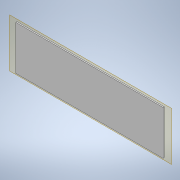
# Autodesk Inventor part: ferrite_layer_dex_laser_cut
Saved by Autodesk Inventor 2020 (Build 240168000, 168)
## iProperties
Created: 2021-01-27
Part Number: ferrite_layer_dex_laser_cut
Material: Generic
Document SubType Name: Modeling
Designer: pduy110
Density: 1 g/cm^3
Appearance: Default
Author: pduy110
Autodesk Inventor part; units mm, degrees
ref_plane "YZ Plane" through (0, 0, 0) normal (1, 0, 0) x (0, 1, 0)
ref_plane "XZ Plane" through (0, 0, 0) normal (0, 1, 0) x (-1, 0, 0)
sketch "ferrite_layer_outline_sketch" plane through (0, 0, 0) normal (0, 0, 1) x (1, 0, 0)
  line L0 (0, 150) -> (1000, 150)
  line L1 (1000, 150) -> (1000, -150)
  line L2 (1000, -150) -> (0, -150)
  line L3 (0, -150) -> (0, 150)
  line L4 (-200, 0) -> (1200, 0) projected
  line L5 (500, 150) -> (500, -150) construction
  line L6 (500, 366.8869) -> (500, -324.3455) construction
  line L7 (20, 109) -> (35, 109)
  line L8 (35, 109) -> (35, -109)
  line L9 (35, -109) -> (20, -109)
  line L10 (20, -109) -> (20, 109)
  line L11 (177.5, -109) -> (177.5, 109)
  line L12 (177.5, 109) -> (192.5, 109)
  line L13 (192.5, 109) -> (192.5, -109)
  line L14 (192.5, -109) -> (177.5, -109)
  line L15 (335, -109) -> (335, 109)
  line L16 (335, 109) -> (350, 109)
  line L17 (350, 109) -> (350, -109)
  line L18 (350, -109) -> (335, -109)
  line L19 (492.5, -109) -> (492.5, 109)
  line L20 (492.5, 109) -> (507.5, 109)
  line L21 (507.5, 109) -> (507.5, -109)
  line L22 (507.5, -109) -> (492.5, -109)
  line L23 (650, -109) -> (650, 109)
  line L24 (650, 109) -> (665, 109)
  line L25 (665, 109) -> (665, -109)
  line L26 (665, -109) -> (650, -109)
  line L27 (807.5, -109) -> (807.5, 109)
  line L28 (807.5, 109) -> (822.5, 109)
  line L29 (822.5, 109) -> (822.5, -109)
  line L30 (822.5, -109) -> (807.5, -109)
  line L31 (965, -109) -> (965, 109)
  line L32 (965, 109) -> (980, 109)
  line L33 (980, 109) -> (980, -109)
  line L34 (980, -109) -> (965, -109)
  line L35 (155, 109) -> (170, 109)
  line L36 (155, -109) -> (155, 109)
  line L37 (170, 109) -> (170, -109)
  line L38 (170, -109) -> (155, -109)
  line L39 (290, 109) -> (305, 109)
  line L40 (290, -109) -> (290, 109)
  line L41 (305, 109) -> (305, -109)
  line L42 (305, -109) -> (290, -109)
  line L43 (425, 109) -> (440, 109)
  line L44 (425, -109) -> (425, 109)
  line L45 (440, 109) -> (440, -109)
  line L46 (440, -109) -> (425, -109)
  line L47 (560, 109) -> (575, 109)
  line L48 (560, -109) -> (560, 109)
  line L49 (575, 109) -> (575, -109)
  line L50 (575, -109) -> (560, -109)
  line L51 (695, 109) -> (710, 109)
  line L52 (695, -109) -> (695, 109)
  line L53 (710, 109) -> (710, -109)
  line L54 (710, -109) -> (695, -109)
  line L55 (830, 109) -> (845, 109)
  line L56 (830, -109) -> (830, 109)
  line L57 (845, 109) -> (845, -109)
  line L58 (845, -109) -> (830, -109)
  line L59 (965, 109) -> (980, 109)
  line L60 (965, -109) -> (965, 109)
  line L61 (980, 109) -> (980, -109)
  line L62 (980, -109) -> (965, -109)
  line L63 (125, -109) -> (125, 109)
  line L64 (125, 109) -> (140, 109)
  line L65 (140, 109) -> (140, -109)
  line L66 (230, -109) -> (230, 109)
  line L67 (230, 109) -> (245, 109)
  line L68 (245, 109) -> (245, -109)
  line L69 (335, -109) -> (335, 109)
  line L70 (335, 109) -> (350, 109)
  line L71 (350, 109) -> (350, -109)
  line L72 (440, -109) -> (440, 109)
  line L73 (440, 109) -> (455, 109)
  line L74 (455, 109) -> (455, -109)
  line L75 (545, -109) -> (545, 109)
  line L76 (545, 109) -> (560, 109)
  line L77 (560, 109) -> (560, -109)
  line L78 (650, -109) -> (650, 109)
  line L79 (650, 109) -> (665, 109)
  line L80 (665, 109) -> (665, -109)
  line L81 (755, -109) -> (755, 109)
  line L82 (755, 109) -> (770, 109)
  line L83 (770, 109) -> (770, -109)
  line L84 (860, -109) -> (860, 109)
  line L85 (860, 109) -> (875, 109)
  line L86 (875, 109) -> (875, -109)
  line L87 (965, -109) -> (965, 109)
  line L88 (965, 109) -> (980, 109)
  line L89 (980, 109) -> (980, -109)
  line L90 (114.5, -109) -> (114.5, 109)
  line L91 (114.5, 109) -> (129.5, 109)
  line L92 (129.5, 109) -> (129.5, -109)
  line L93 (129.5, -109) -> (114.5, -109)
  line L94 (209, -109) -> (209, 109)
  line L95 (209, 109) -> (224, 109)
  line L96 (224, 109) -> (224, -109)
  line L97 (224, -109) -> (209, -109)
  line L98 (303.5, -109) -> (303.5, 109)
  line L99 (303.5, 109) -> (318.5, 109)
  line L100 (318.5, 109) -> (318.5, -109)
  line L101 (318.5, -109) -> (303.5, -109)
  line L102 (398, -109) -> (398, 109)
  line L103 (398, 109) -> (413, 109)
  line L104 (413, 109) -> (413, -109)
  line L105 (413, -109) -> (398, -109)
  line L106 (492.5, -109) -> (492.5, 109)
  line L107 (492.5, 109) -> (507.5, 109)
  line L108 (507.5, 109) -> (507.5, -109)
  line L109 (507.5, -109) -> (492.5, -109)
  line L110 (587, -109) -> (587, 109)
  line L111 (587, 109) -> (602, 109)
  line L112 (602, 109) -> (602, -109)
  line L113 (602, -109) -> (587, -109)
  line L114 (681.5, -109) -> (681.5, 109)
  line L115 (681.5, 109) -> (696.5, 109)
  line L116 (696.5, 109) -> (696.5, -109)
  line L117 (696.5, -109) -> (681.5, -109)
  line L118 (776, -109) -> (776, 109)
  line L119 (776, 109) -> (791, 109)
  line L120 (791, 109) -> (791, -109)
  line L121 (791, -109) -> (776, -109)
  line L122 (870.5, -109) -> (870.5, 109)
  line L123 (870.5, 109) -> (885.5, 109)
  line L124 (885.5, 109) -> (885.5, -109)
  line L125 (885.5, -109) -> (870.5, -109)
  line L126 (965, -109) -> (965, 109)
  line L127 (965, 109) -> (980, 109)
  line L128 (980, 109) -> (980, -109)
  line L129 (980, -109) -> (965, -109)
  point P0 (0, 0)
  point P1 (0, 0)
  point P2 (0, 0)
  point P3 (0, 0)
  point P4 (20, 0)
  point P5 (177.5, 0)
  point P6 (335, 0)
  point P7 (492.5, 0)
  point P8 (650, 0)
  point P9 (807.5, 0)
  point P10 (965, 0)
  point P11 (155, 0)
  point P12 (290, 0)
  point P13 (425, 0)
  point P14 (560, 0)
  point P15 (695, 0)
  point P16 (830, 0)
  point P17 (965, 0)
  point P18 (125, 0)
  point P19 (230, 0)
  point P20 (335, 0)
  point P21 (440, 0)
  point P22 (545, 0)
  point P23 (650, 0)
  point P24 (755, 0)
  point P25 (860, 0)
  point P26 (965, 0)
  point P27 (114.5, 0)
  point P28 (209, 0)
  point P29 (303.5, 0)
  point P30 (398, 0)
  point P31 (492.5, 0)
  point P32 (587, 0)
  point P33 (681.5, 0)
  point P34 (776, 0)
  point P35 (870.5, 0)
  point P36 (965, 0)
  dimension "d0" = 1000
  dimension "d1" = 300
  dimension "d63" = 20
  dimension "d64" = 218
  dimension "d65" = 15
  dimension "d68" = 157.5
  dimension "d75" = 135
  dimension "d82" = 105
  dimension "d89" = 94.5
  constraints: 258 end point, 6 horizontal, 4 collinear, 4 midpoint, 4 parallel, 3 coincident, 3 point on line, 2 perpendicular, 275 other
  measures "d0" distance between parallel lines of L1 L3
  measures "d1" distance between parallel lines of L2 L0
  measures "d63" distance between parallel lines of L10 L3
  measures "d64" distance between parallel lines of L9 L7
  measures "d65" distance between parallel lines of L10 L8
  measures "d68" distance of L9.end L11.start
  measures "d75" distance of L7.start L35.start
  measures "d82" distance of L9.end L63.start
  measures "d89" distance of L7.end L91.end
extrude "Extrusion8" add sketch "ferrite_layer_outline_sketch" along normal blind 8
ref_plane "acrylic_sheet_plane" through (0, 0, 8) normal (0, 0, 1) x (1, 0, 0)
sketch "Sketch4" plane through (0, 0, 8) normal (0, 0, 1) x (1, 0, 0)
  line L0 (20, 109) -> (35, 109)
  line L1 (35, 109) -> (35, -109)
  line L2 (35, -109) -> (20, -109)
  line L3 (20, -109) -> (20, 109)
  line L4 (-12.6534, 0) -> (47.471, 0)
  line L5 (0, 150) -> (0, -150) projected
  line L6 (1000, 150) -> (0, 150) projected
  line L7 (0, -150) -> (1000, -150) projected
  point P0 (0, 0)
  point P1 (20, 0)
  point P2 (0, 0)
  point P3 (500, 150)
  point P4 (500, -150)
  dimension "d43" = 15
  dimension "d44" = 218
  dimension "d45" = 20
  constraints: 10 end point, 4 midpoint, 2 horizontal, 2 parallel, 2 point on line, 1 perpendicular
  measures "d43" distance between parallel lines of L1 L3
  measures "d44" distance between parallel lines of L2 L0
  measures "d45" distance between parallel lines of L5 L3
extrude "Extrusion9" [suppressed]
pattern_linear "Rectangular Pattern1" [suppressed]
pattern_linear "Rectangular Pattern2" [suppressed]
pattern_linear "Rectangular Pattern3" [suppressed]
pattern_linear "pattern_test_#_of_ferrites" [suppressed]
equation "\"d0\" = track_length"
equation "\"d1\" = track_width"
equation "\"d63\" = gap_distance"
equation "\"d64\" = ferrite_length"
equation "\"d65\" = ferrite_width"
equation "\"d43\" = ferrite_width"
equation "\"d44\" = ferrite_length"
equation "\"d45\" = gap_distance"
equation "\"d50\" = parameter_5"
equation "\"d62\" = test_parameter_5"
equation "\"track_length\" = 1000"
equation "\"track_width\" = 300"
equation "\"gap_distance\" = 20"
equation "\"ferrite_length\" = 218"
equation "\"ferrite_width\" = 15"
equation "\"ferrite_height\" = 8"
equation "\"acrylic_sheet_8mm\" = 8"
equation "\"parameter_5\" = 94.5"
equation "\"test_parameter_5\" = 67.5"
body "Solid8"
